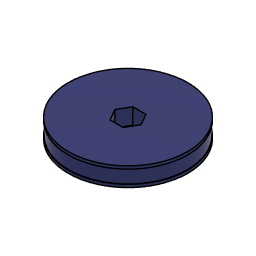
kolo1 v3 (Autodesk Fusion 360 design; units mm, degrees)
Autodesk Fusion 360 part; units mm, degrees
sketch "spodek" plane through (0, 0, 0) normal (0, 1, 0) x (1, 0, 0)
  circle A0 centre (0, 0) radius 31.75
  circle A1 centre (0, 0) radius 2.1
  dimension "d1" = 63.5
  dimension "d2" = 4.2
  constraint coincident A0.centre A1.centre
  measures "d1" diameter of A0
  measures "d2" diameter of A1
extrude "Extrude1" add sketch "spodek" along normal blind 1.5
sketch "prostredek" plane through (0, 1.5, 0) normal (0, 1, 0) x (-1, 0, 0)
  circle A0 centre (0, 0) radius 2.1
  circle A1 centre (0, 0) radius 31.75
  circle A2 centre (0, 0) radius 31.5
  line L0 (3.493, -6.05) -> (6.9859, 0)
  line L1 (6.9859, 0) -> (3.493, 6.05)
  line L2 (3.493, 6.05) -> (-3.493, 6.05)
  line L3 (-3.493, 6.05) -> (-6.9859, 0)
  line L4 (-6.9859, 0) -> (-3.493, -6.05)
  line L5 (-3.493, -6.05) -> (3.493, -6.05)
  dimension "d5" = -0.25
  dimension "d6" = 6.05
  constraint coincident A0.centre A1.centre
  measures "d6" distance of A0.centre L5
extrude "Extrude2" add sketch "prostredek" along normal blind 7 contours A2
sketch "Sketch3" plane through (0, 8.5, 0) normal (0, 1, 0) x (-1, 0, 0)
  line L0 (3.493, -6.05) -> (-3.493, -6.05)
  line L1 (-3.493, -6.05) -> (-6.9859, 0)
  line L2 (-6.9859, 0) -> (-3.493, 6.05)
  line L3 (-3.493, 6.05) -> (3.493, 6.05)
  line L4 (3.493, 6.05) -> (6.9859, 0)
  line L5 (6.9859, 0) -> (3.493, -6.05)
  line L6 (-6.9859, 0) -> (-3.493, 6.05)
  line L7 (-3.493, -6.05) -> (-6.9859, 0)
  line L8 (3.493, -6.05) -> (-3.493, -6.05)
  line L9 (6.9859, 0) -> (3.493, -6.05)
  line L10 (-3.493, 6.05) -> (3.493, 6.05)
  circle A0 centre (0, 0) radius 31.75
extrude "Extrude3" add sketch "Sketch3" along normal blind 1.5
